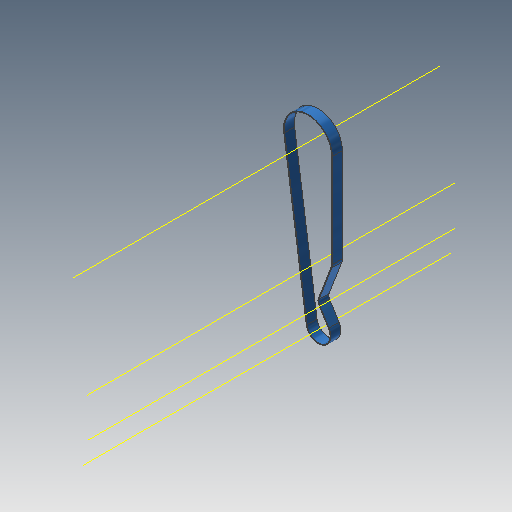
# Autodesk Inventor part: 歯付きベルト
Saved by Autodesk Inventor 2019.4 (Build 234330000, 330)
## iProperties
Created: 2019-11-13
Part Number: 歯付きベルト
Material: Rubber
Document SubType Name: Modeling
Designer: y6tada
Density: 0.93 g/cm^3
Appearance: シアン
Mass: 1.56777 g
Surface Area: 60.4068 cm^2
Volume: 1.68577 cm^3
CustomPartVersion: 1
Author: y6tada
Autodesk Inventor part; units mm, degrees
sketch "スケッチ パス" plane through (0, 0, 0) normal (0, 0, 1) x (1, 0, 0)
  arc A0 (19.09858, 0.022721) -> (-18.901655, -2.735635) centre (0, 0) ccw
  arc A1 (18.716428, -76.913324) -> (19.18706, -74.351396) centre (12.025093, -74.359916) ccw
  arc A2 (8.519671, -103.634445) -> (8.887698, -107.441661) centre (12.537104, -105.167493) ccw
  arc A3 (-1.049291, -126.085154) -> (16.506016, -119.666943) centre (8.401537, -124.717337) ccw
  line L0 (-1.049291, -126.085154) -> (-18.901655, -2.735635)
  line L1 (19.09858, 0.022721) -> (19.18706, -74.351396)
  line L2 (18.716428, -76.913324) -> (8.519671, -103.634445)
  line L3 (8.887698, -107.441661) -> (16.506016, -119.666943)
  constraints: 8 end point, 6 point on circle, 3 centre point, 3 other
ref_plane "断面平面" through (-18.901655, -2.735635, 0) normal (0.1432375, -0.9896883, 0) x (0, 0, 1)
ref_plane "作業平面2" through (0, 0, 0) normal (-1, 0, 0) x (0, 0, 1)
ref_plane "作業平面3" through (8.401537, -124.717337, 0) normal (-0.4316004, 0.9020649, 0) x (0, 0, 1)
ref_plane "作業平面4" through (12.025093, -74.359916, 0) normal (0.0892463, 0.9960096, 0) x (0, 0, 1)
sketch "断面" plane through (-18.901655, -2.735635, 0) normal (0.1432375, -0.9896883, 0) x (0, 0, 1)
  line L0 (-4, 0.3) -> (4, 0.3)
  line L1 (4, 0.3) -> (4, -0.3)
  line L2 (4, -0.3) -> (-4, -0.3)
  line L3 (-4, -0.3) -> (-4, 0.3)
  line L4 (-4, 0) -> (4, 0) construction
  point P0 (0, 0)
  point P1 (0, 0)
  dimension "d0" = 8
  dimension "d4" = 0.3
  dimension "d5" = 0.3
  constraints: 10 end point, 3 midpoint, 2 parallel, 1 coincident, 1 horizontal, 1 perpendicular, 1 other
  measures "d0" distance between parallel lines of L1 L3
  measures "d4" distance between parallel lines of L2 L4
  measures "d5" distance between parallel lines of L4 L0
sweep "ベルト" add profiles "断面" path "スケッチ パス"
equation "\"d4\" = da_a"
equation "\"d5\" = da_a2"
equation "\"da_B\" = 6"
equation "\"da_pb\" = 2.5"
equation "\"da_L\" = 345.26878"
equation "\"da_a\" = 0.3"
equation "\"da_S\" = 1.5"
equation "\"da_Beta\" = 20deg"
equation "\"da_Ht\" = 0.7"
equation "\"da_H\" = 1.3"
equation "\"da_a2\" = 0.3"
body "Solid1"
